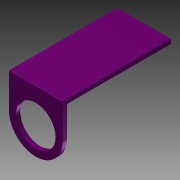
# Autodesk Inventor part: Dudukan Proximity V2
Saved by Autodesk Inventor 2015 (Build 190159000, 159)
## iProperties
Created: 2015-01-10
Part Number: Dudukan Proximity V2
Material: Generic
Document SubType Name: Modeling
Designer: Rafi Kurnia Putra
Density: 1 g/cm^3
Appearance: Smooth - Purple
Author: Rafi Kurnia Putra
Autodesk Inventor part; units mm, degrees
ref_plane "YZ Plane" through (0, 0, 0) normal (1, 0, 0) x (0, 1, 0)
ref_plane "XZ Plane" through (0, 0, 0) normal (0, 1, 0) x (-1, 0, 0)
ref_plane "XY Plane" through (0, 0, 0) normal (0, 0, 1) x (1, 0, 0)
sketch "Sketch1" plane through (0, 0, 0) normal (0, 0, 1) x (1, 0, 0)
  circle A0 centre (0, 15.825) radius 9.125
  line L0 (-12.375, 0) -> (12.375, 0)
  arc A1 (12.375, 15.825) -> (-12.375, 15.825) centre (0, 15.825) ccw
  line L1 (12.375, 0) -> (12.375, 15.825)
  line L2 (-12.375, 0) -> (-12.375, 15.825)
  point P0 (0, 0)
  point P1 (0, 0)
  point P2 (0, 0)
  point P3 (0, 3.45)
  dimension "d28" = 18.25
  dimension "d29" = 24.75
  dimension "d30" = 24.75
  dimension "d31" = 3.45
  constraints: 6 end point, 3 point on circle, 2 centre point, 2 coincident, 2 midpoint, 2 tangent, 1 horizontal
  measures "d28" diameter of A0
  measures "d29" diameter of A1
  measures "d30" distance of L0.start L0.end
  measures "d31" distance of point (0, 0) point (0, 3.45)
sketch "Sketch2" plane through (0, 0, 0) normal (0, 1, 0) x (-1, 0, 0)
  line L0 (12.375, 0) -> (-12.375, 0)
  line L1 (-12.375, 0) -> (-12.375, -50)
  line L2 (-12.375, -50) -> (12.375, -50)
  line L3 (12.375, -50) -> (12.375, 0)
  point P0 (0, 0)
  point P1 (-12.375, 0)
  dimension "d5" = 24.75
  dimension "d10" = 50
  constraints: 8 end point, 2 parallel, 1 horizontal, 1 perpendicular
  measures "d5" distance of L2.end L1.end
  measures "d10" distance of L2.end L0.start
extrude "Extrusion4" add sketch "Sketch2" along normal blind 2
extrude "Extrusion5" add sketch "Sketch1" against normal blind 2
fillet "Fillet1" radius 0.5 2 edges at (0, 0, 0) (0, 2, -2)
body "Solid3"
